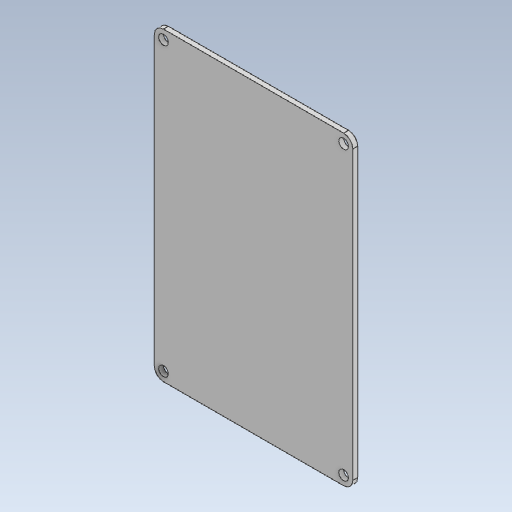
# Autodesk Inventor part: MainBoard
Saved by Autodesk Inventor 2020.4 (Build 244396000, 396)
## iProperties
Created: 2022-01-10
Part Number: MainBoard
Material: 一般
Document SubType Name: Modeling
Designer: Masato Kubotera
Density: 1 g/cm^3
Appearance: 既定
Author: Masato Kubotera
Autodesk Inventor part; units mm, degrees
ref_plane "YZ Plane" through (0, 0, 0) normal (1, 0, 0) x (0, 1, 0)
ref_plane "XZ Plane" through (0, 0, 0) normal (0, 1, 0) x (-1, 0, 0)
ref_plane "XY Plane" through (0, 0, 0) normal (0, 0, 1) x (1, 0, 0)
derived "Cockpit_bottom_frame.ipt"
sketch "スケッチ1" plane through (0, 0, 0) normal (0, 1, 0) x (-1, 0, 0)
  line L0 (-60, 36) -> (60, 36) construction
  line L1 (60, 36) -> (60, -36) construction
  line L2 (60, -36) -> (-60, -36) construction
  line L3 (-60, -36) -> (-60, 36) construction
  line L4 (-60, 36) -> (60, -36) construction
  line L5 (60, 36) -> (-60, -36) construction
  line L6 (-52.5, 6) -> (52.5, 6) construction
  line L7 (52.5, 6) -> (52.5, 1) construction
  line L8 (52.5, 1) -> (-52.5, 1) construction
  line L9 (-52.5, 1) -> (-52.5, 6) construction
  line L10 (-52.5, 6) -> (52.5, 1) construction
  line L11 (52.5, 6) -> (-52.5, 1) construction
  line L12 (0, 36) -> (0, -36) construction
  line L13 (-57.5, 33.5) -> (-52.5, 33.5) construction
  line L14 (-52.5, 33.5) -> (-52.5, -33.5) construction
  line L15 (-52.5, -33.5) -> (-57.5, -33.5) construction
  line L16 (-57.5, -33.5) -> (-57.5, 33.5) construction
  line L17 (-57.5, 33.5) -> (-52.5, -33.5) construction
  line L18 (-52.5, 33.5) -> (-57.5, -33.5) construction
  line L19 (-55, 36) -> (-60, 31)
  line L20 (-60, 0) -> (60, 0) construction
  line L21 (-46.5, 41) -> (32.5, 41) construction
  line L22 (32.5, 41) -> (32.5, 11) construction
  line L23 (32.5, 11) -> (-46.5, 11) construction
  line L24 (-46.5, 11) -> (-46.5, 41) construction
  line L25 (-46.5, 41) -> (32.5, 11) construction
  line L26 (32.5, 41) -> (-46.5, 11) construction
  line L27 (-55, -36) -> (-60, -31)
  line L28 (-60, 31) -> (-60, -31)
  line L29 (55, -36) -> (60, -31)
  line L30 (-52.5, -28.5) -> (52.5, -28.5) construction
  line L31 (52.5, -28.5) -> (52.5, -33.5) construction
  line L32 (52.5, -33.5) -> (-52.5, -33.5) construction
  line L33 (-52.5, -33.5) -> (-52.5, -28.5) construction
  line L34 (-52.5, -28.5) -> (52.5, -33.5) construction
  line L35 (52.5, -28.5) -> (-52.5, -33.5) construction
  line L36 (-25, -28.5) -> (-25, -33.5) construction
  line L37 (-55, -33.5) -> (-55, 33.5) construction
  line L38 (-57.5, 12.5) -> (-52.5, 12.5) construction
  line L39 (-57.55, 12.55) -> (-52.45, 12.55)
  line L40 (-52.45, 12.55) -> (-52.45, -12.55)
  line L41 (-52.45, -12.55) -> (-57.55, -12.55)
  line L42 (-57.55, -12.55) -> (-57.55, 12.55)
  line L43 (-57.55, 12.55) -> (-52.45, -12.55) construction
  line L44 (-52.45, 12.55) -> (-57.55, -12.55) construction
  arc A0 (-52.45, 11.0651) -> (-53.9349, 12.55) centre (-53.1925, 11.8075) ccw
  circle A1 centre (-55, 20) radius 1.6
  circle A2 centre (-55, -20) radius 1.6
  arc A3 (-53.9349, -12.55) -> (-52.45, -11.0651) centre (-53.1925, -11.8075) ccw
  line L45 (-57.5, -12.5) -> (-52.5, -12.5) construction
  arc A4 (-56.0651, 12.55) -> (-57.55, 11.0651) centre (-56.8075, 11.8075) ccw
  arc A5 (-57.55, -11.0651) -> (-56.0651, -12.55) centre (-56.8075, -11.8075) ccw
  line L46 (-52.5, -31) -> (52.5, -31) construction
  line L47 (-25.05, -33.5) -> (-25.05, -28.45)
  line L48 (-25.05, -28.45) -> (25.05, -28.45)
  circle A6 centre (-32.5, -31) radius 1.6
  circle A7 centre (32.5, -31) radius 1.6
  line L49 (25, -28.5) -> (25, -33.5) construction
  line L50 (52.5, 33.5) -> (57.5, 33.5) construction
  line L51 (57.5, 33.5) -> (57.5, -33.5) construction
  line L52 (57.5, -33.5) -> (52.5, -33.5) construction
  line L53 (52.5, -33.5) -> (52.5, 33.5) construction
  line L54 (52.5, 33.5) -> (57.5, -33.5) construction
  line L55 (57.5, 33.5) -> (52.5, -33.5) construction
  line L56 (52.5, 0) -> (57.5, 0) construction
  line L57 (52.5, -12.5) -> (57.5, -12.5) construction
  line L58 (55, -33.5) -> (55, 33.5) construction
  circle A8 centre (55, -20) radius 1.6
  line L59 (60, -12.55) -> (52.45, -12.55)
  line L60 (52.45, -12.55) -> (52.45, 12.55)
  arc A9 (52.45, -11.0651) -> (53.9349, -12.55) centre (53.1925, -11.8075) ccw
  line L61 (52.5, 12.5) -> (57.5, 12.5) construction
  circle A10 centre (55, 20) radius 1.6
  line L62 (60, 12.55) -> (52.45, 12.55)
  arc A11 (53.9349, 12.55) -> (52.45, 11.0651) centre (53.1925, 11.8075) ccw
  arc A12 (-23.5651, -28.45) -> (-25.05, -29.9349) centre (-24.3075, -29.1925) ccw
  arc A13 (25.05, -29.9349) -> (23.5651, -28.45) centre (24.3075, -29.1925) ccw
  circle A14 centre (-55, 20) radius 3
  circle A15 centre (-32.5, -31) radius 3
  circle A16 centre (-55, -20) radius 3
  circle A17 centre (32.5, -31) radius 3
  line L63 (-25.05, -33.5) -> (-27.55, -36)
  line L64 (-55, -36) -> (-27.55, -36)
  line L65 (25.05, -33.5) -> (25.05, -28.45)
  line L66 (25.05, -33.5) -> (27.55, -36)
  line L67 (55, -36) -> (27.55, -36)
  line L68 (25.05, 6.05) -> (-25.05, 6.05)
  line L69 (-25.05, 6.05) -> (-25.05, 0.95)
  line L70 (-25.05, 0.95) -> (25.05, 0.95)
  line L71 (25.05, 0.95) -> (25.05, 6.05)
  line L72 (25.05, 6.05) -> (-25.05, 0.95) construction
  line L73 (-25.05, 6.05) -> (25.05, 0.95) construction
  line L74 (-25, 6) -> (-25, 1) construction
  arc A18 (-23.5651, 6.05) -> (-25.05, 4.5651) centre (-24.3075, 5.3075) ccw
  line L75 (52.5, 3.5) -> (-52.5, 3.5) construction
  circle A19 centre (-32.5, 3.5) radius 1.6
  line L76 (25, 6) -> (25, 1) construction
  arc A20 (25.05, 4.5651) -> (23.5651, 6.05) centre (24.3075, 5.3075) ccw
  circle A21 centre (32.5, 3.5) radius 1.6
  arc A22 (-25.05, 2.4349) -> (-23.5651, 0.95) centre (-24.3075, 1.6925) ccw
  arc A23 (23.5651, 0.95) -> (25.05, 2.4349) centre (24.3075, 1.6925) ccw
  line L77 (60, 31) -> (60, 12.55)
  line L78 (60, -12.55) -> (60, -31)
  circle A24 centre (-32.5, 3.5) radius 3
  circle A25 centre (55, -20) radius 3
  circle A26 centre (55, 20) radius 3
  circle A27 centre (32.5, 3.5) radius 3
  line L79 (60, 31) -> (60, 36)
  line L80 (18, 36) -> (-55, 36)
  line L81 (60, 36) -> (55, 41)
  line L82 (55, 41) -> (50, 41)
  line L83 (50, 41) -> (50, 36)
  line L84 (50, 36) -> (39, 36)
  line L85 (39, 36) -> (39, 41)
  line L86 (39, 41) -> (29, 41)
  line L87 (29, 41) -> (29, 36)
  line L88 (29, 36) -> (18, 36)
  line L89 (18, 36) -> (18, 36)
  circle A28 centre (-45, 3.5) radius 1.75
  line L90 (34, 41) -> (34, 36) construction
  line L91 (37.9, -7.85) -> (47.1, -7.85) construction
  line L92 (47.1, -7.85) -> (47.1, -21.65) construction
  line L93 (47.1, -21.65) -> (37.9, -21.65) construction
  line L94 (37.9, -21.65) -> (37.9, -7.85) construction
  line L95 (37.9, -7.85) -> (47.1, -21.65) construction
  line L96 (47.1, -7.85) -> (37.9, -21.65) construction
  line L97 (37.2, -7.2) -> (47.8, -7.2) construction
  line L98 (47.8, -7.2) -> (47.8, -22.3) construction
  line L99 (47.8, -22.3) -> (37.2, -22.3) construction
  line L100 (37.2, -22.3) -> (37.2, -7.2) construction
  line L101 (37.2, -7.2) -> (47.8, -22.3) construction
  line L102 (47.8, -7.2) -> (37.2, -22.3) construction
  line L103 (42.5, -7.2) -> (42.5, -22.3) construction
  line L104 (47.8, -14.75) -> (37.2, -14.75) construction
  line L105 (38.6349, -7.15) -> (46.3651, -7.15)
  line L106 (37.15, -8.6349) -> (37.15, -20.8651)
  line L107 (39.3349, -7.8) -> (45.6651, -7.8)
  line L108 (37.85, -9.2849) -> (37.85, -20.2151)
  arc A29 (38.6349, -7.15) -> (37.15, -8.6349) centre (37.8925, -7.8925) ccw
  arc A30 (39.3349, -7.8) -> (37.85, -9.2849) centre (38.5925, -8.5425) ccw
  arc A31 (47.85, -8.6349) -> (46.3651, -7.15) centre (47.1075, -7.8925) ccw
  arc A32 (47.15, -9.2849) -> (45.6651, -7.8) centre (46.4075, -8.5425) ccw
  line L109 (38.6349, -22.35) -> (46.3651, -22.35)
  line L110 (39.3349, -21.7) -> (45.6651, -21.7)
  arc A33 (37.15, -20.8651) -> (38.6349, -22.35) centre (37.8925, -21.6075) ccw
  arc A34 (37.85, -20.2151) -> (39.3349, -21.7) centre (38.5925, -20.9575) ccw
  arc A35 (46.3651, -22.35) -> (47.85, -20.8651) centre (47.1075, -21.6075) ccw
  arc A36 (45.6651, -21.7) -> (47.15, -20.2151) centre (46.4075, -20.9575) ccw
  line L111 (47.85, -8.6349) -> (47.85, -20.8651)
  line L112 (47.15, -9.2849) -> (47.15, -20.2151)
  line L113 (-47.5, -3.5) -> (12.5, -3.5)
  line L114 (12.5, -3.5) -> (12.5, -23.5)
  line L115 (12.5, -23.5) -> (-47.5, -23.5)
  line L116 (-47.5, -23.5) -> (-47.5, -3.5)
  line L117 (-47.5, -3.5) -> (12.5, -23.5) construction
  line L118 (12.5, -3.5) -> (-47.5, -23.5) construction
  point P0 (0, 0)
  point P1 (0, 3.5)
  point P2 (-55, 0)
  point P3 (-55, 0)
  point P4 (-7, 26)
  point P5 (0, -31)
  point P6 (0, 3.5)
  point P7 (42.5, -14.75)
  point P8 (37.15, -7.15)
  point P9 (37.85, -7.8)
  point P10 (-17.5, -13.5)
sketch "スケッチ2" plane through (0, 0, -33.5) normal (0, 0, 1) x (1, 0, 0)
  line L0 (52.5, -110.5) -> (52.5, 0)
  line L1 (-52.5, 0) -> (-52.5, -110.5)
  line L2 (-52.5, -110.5) -> (52.5, 0) construction
  line L3 (52.5, -110.5) -> (-52.5, 0) construction
  line L4 (-25, 0) -> (-25, 5)
  line L5 (-25, 5) -> (25, 5)
  line L6 (0, -115.5) -> (0, 5) construction
  line L7 (-52.5, -55.25) -> (52.5, -55.25) construction
  arc A0 (-27.1, 0) -> (-25, 0) centre (-26.05, 0) ccw
  line L8 (25, 0) -> (25, 5)
  arc A1 (25, 0) -> (27.1, 0) centre (26.05, 0) ccw
  arc A2 (-25, -110.5) -> (-27.1, -110.5) centre (-26.05, -110.5) ccw
  line L9 (-25, -110.5) -> (-25, -115.5)
  line L10 (-25, -115.5) -> (25, -115.5)
  line L11 (25, -110.5) -> (25, -115.5)
  arc A3 (27.1, -110.5) -> (25, -110.5) centre (26.05, -110.5) ccw
  line L12 (-52.5, 0) -> (-27.1, 0)
  line L13 (52.5, 0) -> (27.1, 0)
  line L14 (-52.5, -110.5) -> (-27.1, -110.5)
  line L15 (52.5, -110.5) -> (27.1, -110.5)
  line L16 (47.5, -5.25) -> (-17.5, -5.25) construction
  line L17 (-17.5, -5.25) -> (-17.5, -105.25) construction
  line L18 (-17.5, -105.25) -> (47.5, -105.25) construction
  line L19 (47.5, -105.25) -> (47.5, -5.25) construction
  line L20 (47.5, -5.25) -> (-17.5, -105.25) construction
  line L21 (-17.5, -5.25) -> (47.5, -105.25) construction
  circle A4 centre (44.5, -8.25) radius 1.6
  line L22 (-14.5, -102.25) -> (44.5, -102.25) construction
  line L23 (44.5, -102.25) -> (44.5, -8.25) construction
  line L24 (44.5, -8.25) -> (-14.5, -8.25) construction
  line L25 (-14.5, -8.25) -> (-14.5, -102.25) construction
  line L26 (-14.5, -102.25) -> (44.5, -8.25) construction
  line L27 (44.5, -102.25) -> (-14.5, -8.25) construction
  line L28 (15, -5.25) -> (15, -105.25) construction
  circle A5 centre (44.5, -102.25) radius 1.6
  circle A6 centre (-14.5, -102.25) radius 1.6
  circle A7 centre (-14.5, -8.25) radius 1.6
  arc A8 (40.5, -5.25) -> (47.5, -12.25) centre (44.5, -8.25) ccw
  arc A9 (47.5, -98.25) -> (40.5, -105.25) centre (44.5, -102.25) ccw
  arc A10 (-10.5, -105.25) -> (-17.5, -98.25) centre (-14.5, -102.25) ccw
  arc A11 (-17.5, -12.25) -> (-10.5, -5.25) centre (-14.5, -8.25) ccw
  line L29 (40.5, -5.25) -> (-10.5, -5.25)
  line L30 (-17.5, -12.25) -> (-17.5, -98.25)
  line L31 (-10.5, -105.25) -> (40.5, -105.25)
  line L32 (47.5, -98.25) -> (47.5, -12.25)
  circle A12 centre (44.5, -8.25) radius 3
  circle A13 centre (44.5, -102.25) radius 3
  circle A14 centre (-14.5, -102.25) radius 3
  circle A15 centre (-14.5, -8.25) radius 3
  point P0 (0, 0)
  point P1 (0, -55.25)
  point P2 (0, -55.25)
  point P3 (15, -55.25)
sketch "スケッチ3" plane through (0, 0, 0) normal (0, 0, 1) x (1, 0, 0)
  circle A0 centre (-14.5, -8.25) radius 1.6 projected
  line L0 (47.5, -5.25) -> (-17.5, -5.25) construction
  line L1 (-17.5, -5.25) -> (-17.5, -105.25) construction
  line L2 (47.5, -105.25) -> (47.5, -5.25) construction
  circle A1 centre (44.5, -8.25) radius 1.6 projected
  line L3 (-17.5, -105.25) -> (47.5, -105.25) construction
  circle A2 centre (-14.5, -102.25) radius 1.6 projected
  circle A3 centre (44.5, -102.25) radius 1.6 projected
  line L4 (-14.5, -5.25) -> (44.5, -5.25)
  line L5 (47.5, -8.25) -> (47.5, -102.25)
  line L6 (44.5, -105.25) -> (-14.5, -105.25)
  line L7 (-17.5, -102.25) -> (-17.5, -8.25)
  line L8 (-17.5, -5.25) -> (47.5, -105.25) construction
  line L9 (47.5, -5.25) -> (-17.5, -105.25) construction
  arc A4 (47.5, -8.25) -> (44.5, -5.25) centre (44.5, -8.25) ccw
  arc A5 (44.5, -105.25) -> (47.5, -102.25) centre (44.5, -102.25) ccw
  arc A6 (-17.5, -102.25) -> (-14.5, -105.25) centre (-14.5, -102.25) ccw
  arc A7 (-14.5, -5.25) -> (-17.5, -8.25) centre (-14.5, -8.25) ccw
  point P0 (0, 0)
  point P1 (15, -55.25)
  dimension "d1" = 3
  constraints: 12 end point, 8 point on circle, 8 point on line, 8 tangent, 4 centre point, 3 equal radius, 2 midpoint, 2 parallel, 1 horizontal, 1 perpendicular
  measures "d1" radius of A4
extrude "押し出し1" add sketch "スケッチ3" along normal blind 1.6
